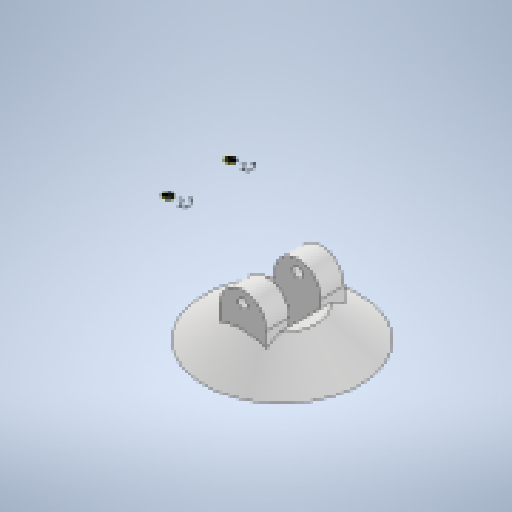
# Autodesk Inventor part: стенд
Saved by Autodesk Inventor 2023 (Build 270158000, 158)
## iProperties
Created: 2024-12-25
Part Number: стенд
Material: Типовые
Document SubType Name: Modeling
Designer: DELL
Density: 1 g/cm^3
Appearance: По умолчанию
Author: DELL
Autodesk Inventor part; units mm, degrees
ref_plane "YZ Plane" through (0, 0, 0) normal (1, 0, 0) x (0, 1, 0)
ref_plane "XZ Plane" through (0, 0, 0) normal (0, 1, 0) x (-1, 0, 0)
ref_plane "XY Plane" through (0, 0, 0) normal (0, 0, 1) x (1, 0, 0)
sketch "Эскиз1" plane through (0, 0, 0) normal (0, 0, 1) x (1, 0, 0)
  line L0 (0, 0) -> (25, 0)
  line L1 (0, 0) -> (0, 18)
  line L2 (0, 18) -> (25, 0)
  line L3 (0, -3.6) -> (0, 21.6) projected
  dimension "d0" = 25
  dimension "d2" = 18
  constraints: 6 end point, 1 horizontal, 1 vertical
  measures "d0" distance of L0.start L0.end
  measures "d2" distance of L0.start L1.end
revolve "Вращение1" add sketch "Эскиз1" angle 360 about axis through (0, -10, 0) along (0, 1, 0)
ref_plane "РабПлоскость1" through (0, 10, 0) normal (0, -1, 0) x (1, 0, 0)
sketch "Эскиз2" plane through (0, 10, 0) normal (0, -1, 0) x (1, 0, 0)
  circle A0 centre (0, 0) radius 11.1111 projected
extrude "Выдавливание1" cut sketch "Эскиз2" against normal blind 10
sketch "Эскиз3" plane through (0, 0, 0) normal (0, 0, 1) x (1, 0, 0)
  line L0 (-7.5, 12.5) -> (-7.5, 0)
  line L1 (-7.5, 0) -> (7.5, 0)
  line L2 (7.5, 0) -> (7.5, 12.5)
  arc A0 (7.5, 12.5) -> (-7.5, 12.5) centre (0, 12.5) ccw
  line L3 (0, 12.5) -> (0, 20) construction
  circle A1 centre (0, 16.25) radius 1.55
  point P0 (0, 0)
  point P1 (0, 0)
  dimension "d10" = 3.1
  constraints: 8 end point, 3 point on circle, 2 centre point, 2 midpoint, 1 coincident, 1 parallel
  measures "d10" diameter of A1
extrude "Выдавливание2" add sketch "Эскиз3" along normal mid plane 25
extrude "Выдавливание3" cut sketch "Эскиз3" along normal mid plane 10
sketch "Эскиз6" plane through (0, 0, 0) normal (0, -1, 0) x (1, 0, 0)
  circle A0 centre (-58.3547, -41.682) radius 1.575 construction
  circle A1 centre (-58.3429, -21.682) radius 1.575 construction
  circle A2 centre (-58.3547, -41.682) radius 1.35
  circle A3 centre (-58.3429, -21.682) radius 1.35
  point P0 (0, 0)
  dimension "d24" = 2.7
  dimension "d25" = 2.7
  constraints: 2 centre point, 2 coincident
  measures "d24" diameter of A2
  measures "d25" diameter of A3
sketch "Эскиз7" plane through (0, 0, 0) normal (0, -1, 0) x (1, 0, 0)
  circle A0 centre (0, -10) radius 1.9
  circle A1 centre (0, 10) radius 1.9
  circle A2 centre (0, 0) radius 25 projected
  line L0 (0, -10) -> (0, 10) construction
  dimension "d29" = 3.8
  dimension "d30" = 20
  constraints: 2 centre point, 2 end point, 1 coincident, 1 equal radius, 1 midpoint
  measures "d29" diameter of A1
  measures "d30" distance of L0.start L0.end
extrude "Выдавливание7" cut sketch "Эскиз7" against normal blind 5 contours A0 | A1
sketch "Эскиз8" plane through (0, 5, 10) normal (0, -1, 0) x (1, 0, 0)
  circle A0 centre (0, 0) radius 1.9 projected
  circle A1 centre (0, -20) radius 1.9 projected
  circle A2 centre (0, 0) radius 1.9 projected
  circle A3 centre (0, 0) radius 1.65
  circle A4 centre (0, -20) radius 1.65
  point P0 (0, -10)
  dimension "d33" = 3.3
  constraints: 2 centre point, 1 equal radius
  measures "d33" diameter of A3
extrude "Выдавливание8" cut sketch "Эскиз8" against normal blind 5 contours A3 | A4
